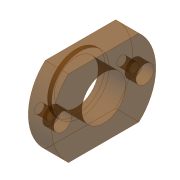
# Autodesk Inventor part: Endpuffer
Saved by Autodesk Inventor 2015 (Build 190159000, 159)
## iProperties
Created: 2015-07-24
Part Number: Endpuffer
Material: PMMA Plastic
Document SubType Name: Modeling
Mass: 7.48184 g
Surface Area: 33.1073 cm^2
Volume: 6.29785 cm^3
Density: 1.188 g/cm^3
Appearance: Polycarbonate - Clear
Autodesk Inventor part; units mm, degrees
ref_plane "YZ Plane" through (0, 0, 0) normal (1, 0, 0) x (0, 1, 0)
ref_plane "XZ Plane" through (0, 0, 0) normal (0, 1, 0) x (-1, 0, 0)
ref_plane "XY Plane" through (0, 0, 0) normal (0, 0, 1) x (1, 0, 0)
sketch "Sketch1" plane through (0, 0, 0) normal (0, 0, 1) x (1, 0, 0)
  line L0 (-2, 10.5) -> (0, 10.5)
  line L1 (0, 10.5) -> (0, 19)
  line L2 (0, 19) -> (8.5, 19)
  line L3 (8.5, 19) -> (8.5, 8)
  line L4 (8.5, 8) -> (-2, 8)
  line L5 (-2, 8) -> (-2, 10.5)
  line L6 (-3.774, 0) -> (9.2238, 0)
  point P0 (0, 0)
  dimension "d0" = 38
  dimension "d1" = 8.5
  dimension "d2" = 10.5
  dimension "d3" = 16
  dimension "d4" = 21
  constraints: 14 end point, 5 perpendicular, 2 horizontal, 2 point on line
  measures "d0" diameter of L2 L6
  measures "d1" distance between parallel lines of L3 L1
  measures "d2" distance between parallel lines of L5 L3
  measures "d3" diameter of L4 L6
  measures "d4" diameter of L0 L6
revolve "Revolution1" add sketch "Sketch1" angle 360 about axis through (-3.774, 0, 0) along (1, 0, 0)
sketch "Sketch2" plane through (8.5, 0, 0) normal (1, 0, 0) x (0, 0, -1)
  line L0 (14, -19) -> (-14, -19)
  line L1 (-14, -19) -> (-14, 19)
  line L2 (-14, 19) -> (14, 19)
  line L3 (14, 19) -> (14, -19)
  line L4 (14, -19) -> (-14, 19) construction
  line L5 (-14, -19) -> (14, 19) construction
  circle A0 centre (0, 0) radius 19 projected
  dimension "d6" = 28
  constraints: 12 end point, 2 midpoint, 2 parallel, 1 horizontal, 1 perpendicular, 1 tangent
  measures "d6" distance between parallel lines of L3 L1
extrude "Extrusion1" cut sketch "Sketch2" against normal blind 10 contours L0 A0 L3 | L0 L1 A0 | A0 L1 L3 | A0 L2 L3 | L1 L2 A0 keep common part
sketch "Sketch3" plane through (8.5, -12.8452, 14) normal (1, 0, 0) x (0, 0, -1)
  point P0 (14, 12.8452)
  point P1 (14, -2.1548)
  point P2 (14, 27.8452)
  dimension "d9" = 30
  dimension "d10" = 15
  constraints: 2 vertical alignment
  measures "d9" distance of point (14, 27.845) point (14, -2.155)
  measures "d10" distance of point (14, 27.845) point (14, 12.845)
hole "Hole1" at (8.5, -15, 0) at (8.5, 15, 0) direction (-1, 0, 0) diameter 3.5 end through all counterbore diameter 6.5 counterbore depth 4
equation "\"d10\" = 0.5 * d9"
body "Solid1"
